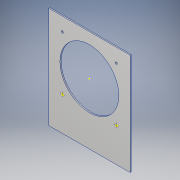
# Autodesk Inventor part: ベアリング板
Saved by Autodesk Inventor 2019 (Build 230136000, 136)
## iProperties
Created: 2020-10-01
Part Number: ベアリング板
Material: アルミニウム 6061
Document SubType Name: Modeling
Designer: Toshihito
Density: 2.7 g/cm^3
Appearance: アルミニウム - フラット
Author: Toshihito
Autodesk Inventor part; units mm, degrees
ref_plane "YZ Plane" through (0, 0, 0) normal (1, 0, 0) x (0, 1, 0)
ref_plane "XZ Plane" through (0, 0, 0) normal (0, 1, 0) x (-1, 0, 0)
ref_plane "XY Plane" through (0, 0, 0) normal (0, 0, 1) x (1, 0, 0)
sketch "スケッチ1" plane through (0, 0, 0) normal (0, 0, 1) x (1, 0, 0)
  line L0 (-100, 100) -> (100, 100)
  line L1 (100, 100) -> (100, -100)
  line L2 (100, -100) -> (-100, -100)
  line L3 (-100, -100) -> (-100, 100)
  line L4 (-100, 100) -> (100, -100) construction
  line L5 (100, 100) -> (-100, -100) construction
  circle A0 centre (0, 0) radius 93.75 construction
  circle A1 centre (-66.2913, 66.2913) radius 2.5
  circle A2 centre (66.2913, 66.2913) radius 2.5
  circle A3 centre (66.2913, -66.2913) radius 2.5
  circle A4 centre (-66.2913, -66.2913) radius 2.5
  dimension "d0" = 200
  dimension "d1" = 200
  dimension "d2" = 187.5
  dimension "d3" = 5
  dimension "d4" = 5
  dimension "d5" = 5
  dimension "d6" = 5
  constraints: 12 end point, 5 centre point, 4 point on circle, 4 point on line, 2 midpoint, 2 parallel, 1 coincident, 1 horizontal, 1 perpendicular
  measures "d0" distance of L1.end L2.end
  measures "d1" distance of L0.end L1.end
  measures "d2" diameter of A0
  measures "d3" diameter of A1
  measures "d4" diameter of A2
  measures "d5" diameter of A3
  measures "d6" diameter of A4
extrude "押し出し1" add sketch "スケッチ1" along normal blind 3
sketch "スケッチ2" plane through (0, 0, 0) normal (0, 0, -1) x (-1, 0, 0)
  circle A0 centre (0, 0) radius 72.5
  dimension "d9" = 145
  constraints: 1 centre point, 1 coincident
  measures "d9" diameter of A0
extrude "押し出し2" cut sketch "スケッチ2" against normal blind 10
sketch "スケッチ3" plane through (0, 0, 3) normal (0, 0, 1) x (1, 0, 0)
  circle A0 centre (-66.2913, -66.2913) radius 2.5 projected
  circle A1 centre (66.2913, -66.2913) radius 2.5 projected
  point P0 (0, 0)
  constraints: 2 coincident
sketch "スケッチ4" plane through (-100, -100, 0) normal (0, -1, 0) x (1, 0, 0)
  line L0 (0, 0) -> (0, 3) projected
  line L1 (200, 0) -> (200, 3) projected
  line L2 (0, 3) -> (200, 3)
  line L3 (200, 3) -> (200, 0)
  line L4 (200, 0) -> (0, 0)
  line L5 (0, 0) -> (0, 3)
  point P0 (100, 0)
  constraints: 8 end point, 2 parallel, 1 horizontal, 1 perpendicular
extrude "押し出し3" add sketch "スケッチ4" along normal blind 50
